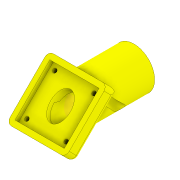
# Autodesk Inventor part: foot3d
Saved by Autodesk Inventor 2020.5 (Build 245400000, 400)
## iProperties
Created: 2022-11-30
Part Number: foot3d
Material: 一般
Document SubType Name: Modeling
Designer: Administrator
Density: 1 g/cm^3
Appearance: 既定「一般マテリアル」(3)
Author: Administrator
Autodesk Inventor part; units mm, degrees
ref_plane "YZ Plane" through (0, 0, 0) normal (1, 0, 0) x (0, 1, 0)
ref_plane "XZ Plane" through (0, 0, 0) normal (0, 1, 0) x (-1, 0, 0)
ref_plane "XY Plane" through (0, 0, 0) normal (0, 0, 1) x (1, 0, 0)
sketch "スケッチ1" plane through (0, 0, 0) normal (0, 0, 1) x (1, 0, 0)
  circle A0 centre (15, 0) radius 10 projected
  circle A1 centre (15, 0) radius 10 projected
  circle A2 centre (15, 0) radius 15 projected
  circle A3 centre (15, 0) radius 16
  circle A4 centre (15, 0) radius 21
  point P0 (0, 0)
  dimension "d0" = 32
  dimension "d1" = 42
  constraints: 2 centre point, 2 coincident, 1 horizontal alignment
  measures "d0" diameter of A3
  measures "d1" diameter of A4
extrude "押し出し1" add sketch "スケッチ1" against normal blind 50 contours A4
sketch "スケッチ2" plane through (15, 0, 0) normal (0, 0, 1) x (1, 0, 0)
  circle A0 centre (0, 0) radius 21 projected
  circle A1 centre (0, 0) radius 16 projected
  circle A2 centre (0, 0) radius 10 projected
  circle A3 centre (0, 0) radius 15 projected
  circle A4 centre (0, 0) radius 10
  circle A5 centre (0, 0) radius 21
  circle A6 centre (0, 0) radius 21 projected
  line L0 (0, -21) -> (0, -24.9885)
  point P0 (-15, 0)
  constraints: 2 centre point, 2 coincident, 2 end point, 1 concentric, 1 horizontal alignment, 1 vertical, 1 vertical alignment, 1 other
extrude "押し出し2" add sketch "スケッチ2" along normal blind 50 contours A0 | A1 | A3
sketch "スケッチ3" plane through (15, 0, -50) normal (0, 0, -1) x (-1, 0, 0)
  circle A0 centre (0, 0) radius 21 projected
  circle A1 centre (0, 0) radius 16 projected
  circle A2 centre (0, 0) radius 21 projected
  circle A3 centre (0, 0) radius 16 projected
  line L0 (0, -21) -> (0.1, -21)
  line L1 (0.1, -21) -> (0.1, -15.9997)
  line L2 (0.1, -15.9997) -> (0, -15.9997)
  line L3 (0, -15.9997) -> (0, -21)
  point P0 (15, 0)
  dimension "d6" = 0.1
  constraints: 8 end point, 2 parallel, 1 horizontal, 1 perpendicular, 1 vertical alignment, 3 other
  measures "d6" distance of L2.end L1.end
extrude "押し出し3" add sketch "スケッチ3" along normal blind 10 contours L3 A1 L1 A0 picked at (0.0889, -17.6665)
sketch "スケッチ4" plane through (15, -21, -50) normal (1, 0, 0) x (0, 0, -1)
  line L0 (0, 5) -> (0, 5.0003) projected
  line L1 (0, 5.0003) -> (0, 5) projected
  line L2 (-50, 5) -> (-50, 37) projected
  line L3 (-100, 0) -> (0, 0) projected
  line L4 (-100, 42) -> (-100, 0) projected
  line L5 (-100, 42) -> (0, 42) projected
  line L6 (0, 0.0002) -> (0, 42) projected
  line L7 (-50, 5) -> (-50, 37) projected
  line L8 (0, 0.0002) -> (-50, 0.0002)
  line L9 (-50, 0.0002) -> (-50, 42)
  line L10 (-50, 42) -> (0, 42)
  line L11 (0, 42) -> (0, 0.0002)
  line L12 (-50, 42) -> (-100, 42)
  line L13 (-100, 42) -> (-100, 0)
  line L14 (-100, 0) -> (-50, 0)
  line L15 (-50, 0) -> (-50, 42)
  line L16 (-50, 42) -> (-120.7107, 112.7107)
  line L17 (-50, 42) -> (50, 42) construction
  line L18 (-50, 11) -> (-50, 31) projected
  line L19 (-50, 31) -> (-81, 0)
  line L20 (-50, 42) -> (-57.0711, 49.0711)
  line L21 (-57.0711, 49.0711) -> (-99.0711, 7.0711)
  line L22 (-99.0711, 7.0711) -> (-92, 0)
  line L23 (-92, 0) -> (-50, 42)
  point P0 (-50, 21)
  dimension "d9" = 100
  dimension "d10" = 135
  dimension "d11" = 10
  constraints: 30 end point, 6 parallel, 3 horizontal, 3 perpendicular, 2 point on line, 1 equal length, 1 midpoint
  measures "d9" distance of L9.end L16.end
  measures "d10" angle of L17 L16
  measures "d11" distance of L9.end L20.end
extrude "押し出し4" cut sketch "スケッチ4" along normal through all both and the other way through all contours L3 L4 L5 L21 L22 | L22 L21 L5 L23
sketch "スケッチ7" plane through (15, 0, 21) normal (0, 0.7071068, 0.7071068) x (1, 0, 0)
  line L0 (-30, 30) -> (30, 30)
  line L1 (30, 30) -> (30, -30)
  line L2 (30, -30) -> (-30, -30)
  line L3 (-30, -30) -> (-30, 30)
  line L4 (-30, 30) -> (30, -30) construction
  line L5 (30, 30) -> (-30, -30) construction
  line L6 (-25, 25) -> (25, 25)
  line L7 (25, 25) -> (25, -25)
  line L8 (25, -25) -> (-25, -25)
  line L9 (-25, -25) -> (-25, 25)
  line L10 (-25, 25) -> (25, -25) construction
  line L11 (25, 25) -> (-25, -25) construction
  line L12 (-20, 20) -> (20, 20)
  line L13 (20, 20) -> (20, -20)
  line L14 (20, -20) -> (-20, -20)
  line L15 (-20, -20) -> (-20, 20)
  line L16 (-20, 20) -> (20, -20) construction
  line L17 (20, 20) -> (-20, -20) construction
  circle A0 centre (-20, 20) radius 2
  circle A1 centre (-20, -20) radius 2
  circle A2 centre (20, 20) radius 2
  circle A3 centre (20, -20) radius 2
  ellipse E0 centre (0, 0) end of major axis (0, -14.1421) minor radius 10 projected
  point P0 (0, 0)
  point P1 (0, 0)
  dimension "d32" = 60
  dimension "d33" = 60
  dimension "d34" = 50
  dimension "d35" = 50
  dimension "d36" = 40
  dimension "d37" = 40
  dimension "d38" = 4
  dimension "d39" = 4
  dimension "d40" = 4
  dimension "d41" = 4
  constraints: 36 end point, 7 midpoint, 6 parallel, 4 centre point, 4 coincident, 3 horizontal, 3 perpendicular, 1 other
  measures "d32" distance of L1.end L2.end
  measures "d33" distance of L0.end L1.end
  measures "d34" distance of L7.end L8.end
  measures "d35" distance of L6.end L7.end
  measures "d36" distance of L13.end L14.end
  measures "d37" distance of L12.end L13.end
  measures "d38" diameter of A0
  measures "d39" diameter of A1
  measures "d40" diameter of A2
  measures "d41" diameter of A3
extrude "押し出し6" add sketch "スケッチ7" along normal mid plane 10 contours L0 L1 L2 L3 | L6 L7 L8 L9 | L12 A2 L13 A3 L14 A1 L15 A0
ref_plane "作業平面1" through (15, -7.0711, 13.9289) normal (0, 0.7071068, 0.7071068) x (1, 0, 0)
sketch "スケッチ11" plane through (15, 3.5355, 24.5355) normal (0, 0.7071068, 0.7071068) x (1, 0, 0)
  circle A0 centre (20, -20) radius 2 projected
  circle A1 centre (-20, -20) radius 2 projected
  circle A2 centre (-20, 20) radius 2 projected
  ellipse E0 centre (0, 0) end of major axis (0, 14.1421) minor radius 10 projected
  circle A3 centre (20, 20) radius 2 projected
  point P0 (-15, 14.8492)
  constraints: 1 other
extrude "押し出し9" cut sketch "スケッチ11" against normal through all contours A0 | A1 | A2 | A3
sketch "スケッチ12" plane through (15, 3.5355, 24.5355) normal (0, 0.7071068, 0.7071068) x (1, 0, 0)
  line L0 (-30, 30) -> (30, 30)
  line L1 (30, 30) -> (30, -30)
  line L2 (30, -30) -> (-30, -30)
  line L3 (-30, -30) -> (-30, 30)
  line L4 (-30, 30) -> (30, -30) construction
  line L5 (30, 30) -> (-30, -30) construction
  line L6 (-25, 25) -> (25, 25)
  line L7 (25, 25) -> (25, -25)
  line L8 (25, -25) -> (-25, -25)
  line L9 (-25, -25) -> (-25, 25)
  line L10 (-25, 25) -> (25, -25) construction
  line L11 (25, 25) -> (-25, -25) construction
  line L12 (-20, 20) -> (20, 20)
  line L13 (20, 20) -> (20, -20)
  line L14 (20, -20) -> (-20, -20)
  line L15 (-20, -20) -> (-20, 20)
  line L16 (-20, 20) -> (20, -20) construction
  line L17 (20, 20) -> (-20, -20) construction
  circle A0 centre (-20, 20) radius 2
  circle A1 centre (-20, -20) radius 2
  circle A2 centre (20, 20) radius 2
  circle A3 centre (20, -20) radius 2
  ellipse E0 centre (0, 0) end of major axis (0, -14.1421) minor radius 10
  point P0 (-15, 14.8492)
  point P1 (0, 0)
  point P2 (0, 0)
  dimension "d56" = 60
  dimension "d57" = 60
  dimension "d58" = 50
  dimension "d59" = 50
  dimension "d60" = 40
  dimension "d61" = 40
  dimension "d62" = 4
  dimension "d63" = 4
  dimension "d64" = 4
  dimension "d65" = 4
  constraints: 36 end point, 7 midpoint, 6 parallel, 4 centre point, 4 coincident, 3 horizontal, 3 perpendicular, 2 other
  measures "d56" distance of L1.end L2.end
  measures "d57" distance of L0.end L1.end
  measures "d58" distance of L7.end L8.end
  measures "d59" distance of L6.end L7.end
  measures "d60" distance of L13.end L14.end
  measures "d61" distance of L12.end L13.end
  measures "d62" diameter of A0
  measures "d63" diameter of A1
  measures "d64" diameter of A2
  measures "d65" diameter of A3
extrude "押し出し10" add sketch "スケッチ12" along normal blind 5 contours L0 L1 L2 L3
sketch "スケッチ13" plane through (15, -3.5355, 17.4645) normal (0, -0.7071068, -0.7071068) x (-1, 0, 0)
  ellipse E0 centre (0, 5) end of major axis (0, -24.6985) minor radius 21 (-11.3358, 30) -> (-18.0167, 20.2577) ccw projected
  line L0 (-11.3358, 30) -> (-30, 30) projected
  line L1 (-30, 30) -> (-30, -30) projected
  line L2 (-30, -30) -> (30, -30) projected
  line L3 (30, -30) -> (30, 30) projected
  line L4 (30, 30) -> (11.3358, 30) projected
  ellipse E1 centre (0, 5) end of major axis (0, -24.6985) minor radius 21 (18.0167, 20.2577) -> (11.3358, 30) ccw projected
  arc A0 (18.7174, 18.4654) -> (18.0167, 20.2577) centre (20, 20) ccw projected
  ellipse E2 centre (0, 5) end of major axis (0, -24.6985) minor radius 21 (-18.7174, 18.4654) -> (18.7174, 18.4654) ccw projected
  arc A1 (-18.0167, 20.2577) -> (-18.7174, 18.4654) centre (-20, 20) ccw projected
  circle A2 centre (20, -20) radius 2 projected
  circle A3 centre (-20, -20) radius 2 projected
  circle A4 centre (-20, 20) radius 2 projected
  circle A5 centre (-20, 20) radius 4
  circle A6 centre (20, 20) radius 4
  circle A7 centre (20, -20) radius 2 projected
  circle A8 centre (20, -20) radius 4
  circle A9 centre (-20, -20) radius 2 projected
  circle A10 centre (-20, -20) radius 4
  point P0 (15, 14.8492)
  point P1 (19.4975, 16.0317)
  point P2 (16.9323, 22.5669)
  dimension "d68" = 8
  dimension "d69" = 8
  dimension "d70" = 8
  dimension "d71" = 8
  constraints: 4 centre point, 4 coincident, 3 other
  measures "d68" diameter of A5
  measures "d69" diameter of A6
  measures "d70" diameter of A8
  measures "d71" diameter of A10
extrude "押し出し11" cut sketch "スケッチ13" along normal blind 50 and the other way blind 5 contours A5 E2 A4 E0 | E0 A1 E2 A5 | A6 E1 A0 E2 | E2 A0 E1 A6 | A8 | A10
fillet "フィレット1" radius 5 8 edges at (15, -24.7487, 38.6777) (45, -3.5355, 17.4645) (-15, -3.5355, 17.4645) (-5.6679, 17.6777, -3.7487) (-15, 22.981, 1.5546) (-15, -19.4454, 43.981) (45, -19.4454, 43.981) (45, 22.981, 1.5546)
